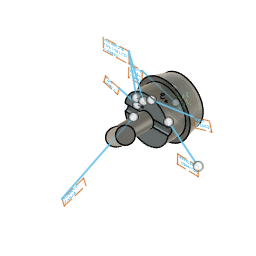
Wireless sthetoscope_ (Autodesk Fusion 360 design; units mm, degrees)
Autodesk Fusion 360 part; units mm, degrees
sketch "Sketch1" plane through (0, 0, 0) normal (0, 1, 0) x (1, 0, 0)
  circle A0 centre (0, 0) radius 25
  dimension "d1" = 50
  constraint coincident A0.centre origin
  measures "d1" diameter of A0
extrude "Extrude1" add sketch "Sketch1" along normal blind 40
sketch "Sketch2" plane through (0, 0, 0) normal (0, -1, 0) x (1, 0, 0)
  circle A0 centre (0, 0) radius 25
ref_plane "WorkPlane1" through (0, 20, 0) normal (0, 1, 0) x (1, 0, 0)
sketch "Sketch3" plane through (0, 20, 0) normal (0, 1, 0) x (1, 0, 0)
  circle A0 centre (0, 0) radius 30
  dimension "d5" = 60
  constraint coincident A0.centre origin
  measures "d5" diameter of A0
loft "Loft1" add profiles "Sketch3" section 1 face at (-6.7759, 40, 1.242) section 2
sketch "Sketch4" plane through (0, 40, 0) normal (0, 1, 0) x (-1, 0, 0)
  circle A0 centre (0, 0) radius 25
  circle A1 centre (0, 0) radius 20
  line L0 (0, 0) -> (0, 38.2916) construction
  line L1 (0, 0) -> (-10, 0)
  arc A2 (0, 38.2916) -> (-10, 0) centre (13.8608, 14.2202) ccw
  line L2 (-10.1114, 28.2518) -> (0, 0)
  dimension "d6" = 40
  dimension "d7" = 10
  constraint concentric A0 A1
  constraint coincident A0.centre A1.centre
  constraint vertical L0
  constraint perpendicular L0 L1
  constraint coincident A2 L2.start
  measures "d6" diameter of A1
  measures "d7" distance of A0.centre L1.end
sketch "Sketch5" plane through (0, 0, 0) normal (1, 0, 0) x (0, 1, 0)
  circle A0 centre (0, 0) radius 4
  dimension "d9" = 8
  constraint coincident A0.centre origin
  measures "d9" diameter of A0
extrude "Extrude2" cut sketch "Sketch5" along normal mid plane 60
sketch "Sketch7" plane through (0, 0, 0) normal (0, -1, 0) x (1, 0, 0)
  circle A0 centre (0, 0) radius 2.5
  dimension "d13" = 5
  constraint coincident A0.centre origin
  measures "d13" diameter of A0
extrude "Extrude3" cut sketch "Sketch7" along normal mid plane 100
sketch "Sketch8" plane through (0, 0, 0) normal (0, -1, 0) x (1, 0, 0)
  circle A0 centre (0, 0) radius 8.1615
  line L0 (0, 0, 0) -> (0, 0, 34.4695)
  line L1 (0, 0, 34.4695) -> (25.5568, 22.0424, 49.8902)
  constraint coincident A0.centre origin
sweep "Sweep1" add profiles "Sketch8" path "Sketch8" along L0 L1 section 1
delete_face "DeleteFace1" 1 faces at (0.0056, 27.7075, 2.5)
sketch "Sketch9" plane through (0, 0, 0) normal (0, 0, 1) x (1, 0, 0)
  circle A0 through (11.7161, 8.2506, 22.8173) (9.4661, 9.5496, 22.8173) (9.4661, 6.9515, 22.8173)
  dimension "d22" = 3
extrude "Extrude4" add sketch "Sketch9" along normal blind 3 contours A0 in plane through (0, 0, 22.8173) normal (0, 0, 1)
sketch "Sketch10" plane through (0, 0, 0) normal (0, -1, 0) x (1, 0, 0)
  line L0 (-12, 12.5) -> (-4, 12.5)
  line L1 (-4, 12.5) -> (-4, 9.5)
  line L2 (-4, 9.5) -> (-12, 9.5)
  line L3 (-12, 9.5) -> (-12, 12.5)
  line L4 (-12, 12.5) -> (-4, 9.5) construction
  line L5 (-4, 12.5) -> (-12, 9.5) construction
  point P0 (-8, 11)
  dimension "d25" = 3
  constraint horizontal L0
  constraint perpendicular L0 L1
  constraint parallel L0 L2
  constraint parallel L1 L3
  constraint coincident L4 P0
  constraint coincident L5 P0
  measures "d25" distance of L0.end L1.end
extrude "Extrude5" cut sketch "Sketch10" against normal blind 2
sketch "Sketch11" plane through (0, 0, 0) normal (0, -1, 0) x (1, 0, 0)
  line L0 (-11, 10) -> (-5, 10)
  line L1 (-5, 10) -> (-5, 12)
  line L2 (-5, 12) -> (-11, 12)
  line L3 (-11, 12) -> (-11, 10)
  line L4 (-11, 10) -> (-5, 12) construction
  line L5 (-5, 10) -> (-11, 12) construction
  point P0 (-8, 11)
  constraint horizontal L0
  constraint perpendicular L0 L1
  constraint parallel L0 L2
  constraint parallel L1 L3
  constraint coincident L4 P0
  constraint coincident L5 P0
extrude "Extrude6" cut sketch "Sketch11" against normal blind 3
sketch "Sketch12" plane through (0, 40, 0) normal (0, 1, 0) x (-1, 0, 0)
  circle A0 centre (0, 0) radius 25
  circle A1 centre (0, 0) radius 23.5
  dimension "d30" = 47
  constraint coincident A0.centre A1.centre
  measures "d30" diameter of A1
extrude "Extrude7" cut sketch "Sketch12" against normal blind 0.2 contours A1
sketch "Sketch13" plane through (0, 0, 0) normal (0, -1, 0) x (1, 0, 0)
  circle A0 centre (-4, 15) radius 1
  circle A1 centre (-11, 15) radius 1
  dimension "d33" = 2
  dimension "d34" = 2
  measures "d33" diameter of A0
  measures "d34" diameter of A1
extrude "Extrude8" cut sketch "Sketch13" against normal blind 1.5
sketch "Sketch14" plane through (0, 0, 0) normal (0, -1, 0) x (1, 0, 0)
  circle A0 centre (-4, 15) radius 0.7049
  circle A1 centre (-11, 15) radius 0.705
  dimension "d37" = 1.41
  measures "d37" diameter of A1
extrude "Extrude9" cut sketch "Sketch14" against normal blind 3
sketch "Sketch15" plane through (0, 0, 0) normal (0, 0, 1) x (1, 0, 0)
  circle A0 through (14.5284, 8.6212, 21.0234) (13.0284, 9.4872, 21.0234) (13.0284, 7.7552, 21.0234)
  dimension "d40" = 2
extrude "Extrude10" cut sketch "Sketch15" against normal blind 1 contours A0 in plane through (0, 0, 21.0234) normal (0, 0, 1)
sketch "Sketch16" plane through (0, 39.8, 0) normal (0, 1, 0) x (-1, 0, 0)
  circle A0 centre (0, 0) radius 23.5
  line L0 (6.0916, -5.9745) -> (44.6424, 6.1108)
  line L1 (44.867, -8.4345) -> (60.4018, -8.1947) construction
  line L2 (60.4018, -8.1947) -> (60.1772, 6.3506) construction
  line L3 (60.1772, 6.3506) -> (44.6424, 6.1108) construction
  line L4 (44.6424, 6.1108) -> (44.867, -8.4345) construction
  dimension "d43" = 3
  constraint coincident L0.end
sketch "Sketch17" plane through (0, 0, 0) normal (0, 1, 0) x (1, 0, 0)
  line L0 (5.7072, -22.366) -> (53.6011, -29.4329)
  line L1 (56.3307, -19.7417) -> (75, -25) construction
  line L2 (75, -25) -> (72.2704, -34.6912) construction
  line L3 (72.2704, -34.6912) -> (53.6011, -29.4329) construction
  line L4 (53.6011, -29.4329) -> (56.3307, -19.7417) construction
  dimension "d44" = 3
  constraint coincident L0.end
sketch "Sketch18" plane through (0, 0, 0) normal (0, -1, 0) x (1, 0, 0)
  line L0 (-10.364, 9.6891) -> (-31.4215, 15.3762)
  line L1 (-49.1101, 12.9436) -> (-33.3605, 8.5013) construction
  line L2 (-33.3605, 8.5013) -> (-31.4215, 15.3762) construction
  line L3 (-31.4215, 15.3762) -> (-47.171, 19.8184) construction
  line L4 (-47.171, 19.8184) -> (-49.1101, 12.9436) construction
  dimension "d45" = 3
  constraint coincident L0.end
sketch "Sketch19" plane through (0, 0, 0) normal (0, -1, 0) x (1, 0, 0)
  line L0 (-11.4815, 16.0174) -> (-20.4373, 57.768)
  line L1 (-20.4373, 57.768) -> (-3.4435, 16.58)
  line L2 (-49.495, 43.9899) -> (-20, 45) construction
  line L3 (-20, 45) -> (-20.4373, 57.768) construction
  line L4 (-20.4373, 57.768) -> (-49.9323, 56.7579) construction
  line L5 (-49.9323, 56.7579) -> (-49.495, 43.9899) construction
  dimension "d46" = 3
  constraint coincident L0.end
sketch "Sketch20" plane through (0, 0, 0) normal (1, 0, 0) x (0, 1, 0)
  line L0 (-15.0143, 10.0119) -> (-97.2588, -30.1968)
  line L1 (-94.5703, -38.6682) -> (-69.693, -30.7729) construction
  line L2 (-69.693, -30.7729) -> (-72.3816, -22.3016) construction
  line L3 (-72.3816, -22.3016) -> (-97.2588, -30.1968) construction
  line L4 (-97.2588, -30.1968) -> (-94.5703, -38.6682) construction
  dimension "d47" = 3
  constraint coincident L0.end
sketch "Sketch21" plane through (0, 0, 0) normal (0, -1, 0) x (1, 0, 0)
  line L0 (25.2413, 10.2779) -> (59.3677, -16.8869)
sketch "Sketch22" plane through (0, 0, 0) normal (0, -1, 0) x (1, 0, 0)
  line L0 (59.2741, -27.1776) -> (35.5501, -26.5067) construction
  line L1 (35.5501, -26.5067) -> (35.8381, -16.3245) construction
  line L2 (35.8381, -16.3245) -> (59.5621, -16.9955) construction
  line L3 (59.5621, -16.9955) -> (59.2741, -27.1776) construction
  dimension "d49" = 3
